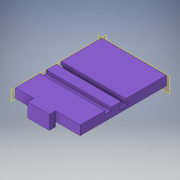
# Autodesk Inventor part: BandSawJigBottomSpiltA-SpiltA
Saved by Autodesk Inventor 2018.2 (Build 222227000, 227)
## iProperties
Created: 2017-12-10
Part Number: BandSawJigBottomSpiltA-SpiltA
Material: LCP Plastic
Document SubType Name: Modeling
Designer: steele
Density: 1.626 g/cm^3
Appearance: Violet
Author: steele
Autodesk Inventor part; units mm, degrees
ref_plane "YZ Plane" through (0, 0, 0) normal (1, 0, 0) x (0, 1, 0)
ref_plane "XZ Plane" through (0, 0, 0) normal (0, 1, 0) x (-1, 0, 0)
sketch "Sketch3" plane through (0, 0, 0) normal (0, 0, 1) x (1, 0, 0)
  line L0 (0, -9.525) -> (9.525, -9.525)
  line L1 (9.525, -9.525) -> (9.525, 0)
  line L2 (0, 0) -> (0, -9.525) construction
  line L3 (0, 0) -> (9.525, 0) construction
  line L4 (0, -9.525) -> (-9.525, -9.525)
  line L5 (-9.525, -9.525) -> (-9.525, 0)
  line L6 (9.525, 0) -> (73.025, 0)
  line L7 (-187.325, 0) -> (-187.325, 19.05)
  line L8 (-187.325, 0) -> (-9.525, 0)
  line L9 (73.025, 0) -> (73.025, 19.05)
  line L10 (73.025, 19.05) -> (-187.325, 19.05)
  dimension "d0" = 9.525
  dimension "d1" = 9.525
  dimension "d6" = 63.5
  dimension "d8" = 19.05
  dimension "d9" = 177.8
  constraints: 22 end point, 4 horizontal, 3 perpendicular, 2 symmetric about line, 1 vertical
  measures "d0" distance of L0.end L1.end
  measures "d1" distance of L0.start L0.end
  measures "d6" distance of L1.end L6.end
  measures "d8" distance of L6.end L9.end
  measures "d9" distance of L7.start L5.end
extrude "Extrusion1" add sketch "Sketch3" along normal mid plane 355.6
sketch "Sketch4" plane through (0, 0, 177.8) normal (0, 0, 1) x (1, 0, 0)
  line L0 (-187.325, 19.05) -> (73.025, 19.05) construction
  line L1 (0, 19.05) -> (0, -9.525) construction
  line L2 (9.525, -9.525) -> (-9.525, -9.525) construction
  line L3 (0, -9.525) -> (-22.225, -9.525)
  line L4 (-22.225, -9.525) -> (-22.225, 19.05)
  line L5 (-22.225, 19.05) -> (0, 19.05)
  line L6 (187.325, 19.05) -> (-73.025, 19.05) construction
  line L7 (0, -9.525) -> (22.225, -9.525)
  line L8 (22.225, -9.525) -> (22.225, 19.05)
  line L9 (0, 19.05) -> (22.225, 19.05)
  point P0 (0, 0)
  dimension "d12" = 22.225
  constraints: 16 end point, 4 point on line, 4 symmetric about line, 2 collinear, 1 midpoint, 1 perpendicular
  measures "d12" distance of L1.end L3.end
extrude "Extrusion2" add sketch "Sketch4" along normal blind 12.7
mirror "Mirror1" about plane through (0, 0, 0) normal (0, 0, 1) of "Extrusion2"
sketch "Sketch6" plane through (-187.325, 0, -177.8) normal (0, -1, 0) x (1, 0, 0)
  line L0 (82.55, 165.1) -> (88.9, 165.1)
  line L1 (88.9, 165.1) -> (88.9, 190.5)
  line L2 (88.9, 190.5) -> (82.55, 190.5)
  line L3 (82.55, 190.5) -> (82.55, 165.1)
  line L4 (82.55, 165.1) -> (88.9, 190.5) construction
  line L5 (88.9, 165.1) -> (82.55, 190.5) construction
  line L6 (177.8, 0) -> (177.8, 355.6) projected
  point P0 (187.325, 177.8)
  point P1 (85.725, 177.8)
  dimension "d16" = 12.7
  dimension "d18" = 6.35
  dimension "d19" = 88.9
  constraints: 12 end point, 2 midpoint, 2 parallel, 1 horizontal, 1 perpendicular
  measures "d16" distance from line of L2 point (85.725, 177.8)
  measures "d18" distance of L1.end L2.end
  measures "d19" distance between parallel lines of L1 L6
extrude "Extrusion3" cut sketch "Sketch6" against normal through all
sketch "Sketch7" plane through (0, 0, 177.8) normal (0, 0, 1) x (1, 0, 0)
  line L0 (-187.325, 19.05) -> (-22.225, 19.05) projected
  line L1 (-161.925, 19.05) -> (-117.475, 19.05)
  line L2 (-117.475, 19.05) -> (-117.475, -3.81)
  line L3 (-117.475, -3.81) -> (-161.925, -3.81)
  line L4 (-161.925, -3.81) -> (-161.925, 19.05)
  line L5 (-187.325, 19.05) -> (-187.325, 0) projected
  point P0 (0, 0)
  dimension "d22" = 44.45
  dimension "d23" = 22.86
  dimension "d24" = 25.4
  constraints: 8 end point, 2 parallel, 1 horizontal, 1 perpendicular, 1 point on line
  measures "d22" distance of L2.end L3.end
  measures "d23" distance of L1.end L2.end
  measures "d24" distance between parallel lines of L4 L5
extrude "Extrusion4" add sketch "Sketch7" along normal blind 12.7
mirror "Mirror2" about plane through (0, 0, 0) normal (0, 0, 1) of "Extrusion4"
sketch "Sketch9" plane through (73.025, 0, 177.8) normal (1, 0, 0) x (0, 0, -1)
  line L0 (355.6, 19.05) -> (0, 19.05) projected
  line L1 (50.8, 19.05) -> (63.5, 19.05)
  line L2 (63.5, 19.05) -> (63.5, 12.7)
  line L3 (63.5, 12.7) -> (50.8, 12.7)
  line L4 (50.8, 12.7) -> (50.8, 19.05)
  line L5 (0, 0) -> (0, 19.05) projected
  point P0 (177.8, 0)
  dimension "d28" = 12.7
  dimension "d29" = 6.35
  dimension "d30" = 50.8
  constraints: 8 end point, 2 parallel, 1 horizontal, 1 perpendicular, 1 point on line
  measures "d28" distance of L2.end L3.end
  measures "d29" distance of L1.end L2.end
  measures "d30" distance between parallel lines of L4 L5
extrude "Extrusion5" cut sketch "Sketch9" against normal through all
mirror "Mirror3" about plane through (0, 0, 0) normal (0, 0, 1) of "Extrusion5"
sketch "Sketch12" plane through (73.025, 0, 177.8) normal (1, 0, 0) x (0, 0, -1)
  line L0 (355.6, 0) -> (0, 0) construction
  line L1 (88.9, 0) -> (88.9, 16.5009) construction
  line L2 (0, 0) -> (0, 19.05) projected
  line L3 (50.8, 19.05) -> (0, 19.05) projected
  line L4 (84.1375, 19.05) -> (84.1375, 12.7)
  line L5 (84.1375, 12.7) -> (80.1624, 12.7)
  line L6 (80.1624, 12.7) -> (80.1624, 6.35)
  line L7 (80.1624, 6.35) -> (88.9, 6.35)
  line L8 (93.6625, 19.05) -> (93.6625, 12.7)
  line L9 (93.6625, 12.7) -> (97.6376, 12.7)
  line L10 (97.6376, 12.7) -> (97.6376, 6.35)
  line L11 (97.6376, 6.35) -> (88.9, 6.35)
  line L12 (84.1375, 19.05) -> (93.6625, 19.05)
  point P0 (177.8, 0)
  dimension "d46" = 88.9
  dimension "d47" = 4.7625
  dimension "d48" = 6.35
  dimension "d49" = 6.35
  dimension "d50" = 8.7376
  constraints: 20 end point, 4 symmetric about line, 3 point on line, 3 vertical, 1 collinear, 1 horizontal, 1 perpendicular
  measures "d46" distance between parallel lines of L1 L2
  measures "d47" distance between parallel lines of L4 L1
  measures "d48" distance of L4.start L4.end
  measures "d49" distance of L5.end L6.end
  measures "d50" distance of L6.end L7.end
extrude "Extrusion8" cut sketch "Sketch12" against normal through all
mirror "Mirror4" about plane through (0, 0, 0) normal (0, 0, 1) of "Extrusion8"
split "Split2" plane through (0, 0, 0) removes the side toward (0, 0, -1)
ref_plane "Work Plane1" through (-60.325, 0, 177.8) normal (1, 0, 0) x (0, 0, -1)
split "Split3" plane through (-60.325, 0, 177.8) removes the side toward (-1, 0, 0)
body "Solid1"
